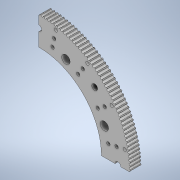
# Autodesk Inventor part: 152ToothBase
Saved by Autodesk Inventor 2020 (Build 240168000, 168)
## iProperties
Created: 2020-01-19
Part Number: 152ToothBase
Material: Generic
Document SubType Name: Modeling
Designer: srini
Density: 1 g/cm^3
Appearance: Default
Author: srini
Autodesk Inventor part; units mm, degrees
ref_plane "YZ Plane" through (0, 0, 0) normal (1, 0, 0) x (0, 1, 0)
ref_plane "XZ Plane" through (0, 0, 0) normal (0, 1, 0) x (-1, 0, 0)
ref_plane "XY Plane" through (0, 0, 0) normal (0, 0, 1) x (1, 0, 0)
sketch "Sketch1" plane through (0, 0, 0) normal (0, 0, 1) x (1, 0, 0)
  circle A0 centre (0, 0) radius 139.485
  dimension "d0" = 278.97
  constraints: 1 centre point, 1 coincident
  measures "d0" diameter of A0
extrude "Extrusion1" add sketch "Sketch1" along normal blind 16
sketch "Sketch2" plane through (0, 0, 16) normal (0, 0, 1) x (1, 0, 0)
  arc A0 (-1.543, 138.9452) -> (1.543, 138.9452) centre (0, 138.9452) ccw
  line L0 (-2.0752, 139.4696) -> (-2.0752, 141.0997)
  line L1 (-2.0752, 141.0997) -> (2.0752, 141.0997)
  line L2 (2.0752, 141.0997) -> (2.0752, 139.4696)
  circle A1 centre (0, 0) radius 139.485 construction
  arc A2 (-1.543, 138.9452) -> (-2.0752, 139.4696) centre (-2.0674, 138.9452) ccw
  arc A3 (2.0752, 139.4696) -> (1.543, 138.9452) centre (2.0674, 138.9452) ccw
  dimension "d3" = 1.543
  dimension "d47" = 2.0828
  constraints: 8 point on circle, 6 end point, 3 centre point, 3 tangent, 2 horizontal alignment, 2 vertical, 1 equal radius, 1 perpendicular, 1 vertical alignment
  measures "d3" radius of A0
extrude "Extrusion2" cut sketch "Sketch2" against normal through all
pattern_circular "Circular Pattern1" count 176 over 360 about axis through (0, 0, 0) along (0, 0, 1) of "Extrusion2"
sketch "Sketch3" plane through (0, 0, 16) normal (0, 0, 1) x (1, 0, 0)
  circle A0 centre (21.06, 105.8758) radius 2.5797
  line L0 (21.06, 105.8758) -> (3.1113, 15.6417) construction
  circle A1 centre (23.5376, 118.3317) radius 2.5797
  circle A2 centre (26.0153, 130.7877) radius 2.5797
  circle A3 centre (-21.06, 105.8758) radius 2.5797
  circle A4 centre (-23.5376, 118.3317) radius 2.5797
  circle A5 centre (-26.0153, 130.7877) radius 2.5797
  circle A6 centre (-59.9738, 89.7571) radius 2.5797
  circle A7 centre (-67.0295, 100.3168) radius 2.5797
  circle A8 centre (-74.0853, 110.8765) radius 2.5797
  circle A9 centre (-89.7571, 59.9738) radius 2.5797
  circle A10 centre (-100.3168, 67.0295) radius 2.5797
  circle A11 centre (-110.8765, 74.0853) radius 2.5797
  circle A12 centre (-105.8758, 21.06) radius 2.5797
  circle A13 centre (-118.3317, 23.5376) radius 2.5797
  circle A14 centre (-130.7877, 26.0153) radius 2.5797
  circle A15 centre (-105.8758, -21.06) radius 2.5797
  circle A16 centre (-118.3317, -23.5376) radius 2.5797
  circle A17 centre (-130.7877, -26.0153) radius 2.5797
  circle A18 centre (-89.7571, -59.9738) radius 2.5797
  circle A19 centre (-100.3168, -67.0295) radius 2.5797
  circle A20 centre (-110.8765, -74.0853) radius 2.5797
  circle A21 centre (-59.9738, -89.7571) radius 2.5797
  circle A22 centre (-67.0295, -100.3168) radius 2.5797
  circle A23 centre (-74.0853, -110.8765) radius 2.5797
  circle A24 centre (-21.06, -105.8758) radius 2.5797
  circle A25 centre (-23.5376, -118.3317) radius 2.5797
  circle A26 centre (-26.0153, -130.7877) radius 2.5797
  circle A27 centre (21.06, -105.8758) radius 2.5797
  circle A28 centre (23.5376, -118.3317) radius 2.5797
  circle A29 centre (26.0153, -130.7877) radius 2.5797
  circle A30 centre (59.9738, -89.7571) radius 2.5797
  circle A31 centre (67.0295, -100.3168) radius 2.5797
  circle A32 centre (74.0853, -110.8765) radius 2.5797
  circle A33 centre (89.7571, -59.9738) radius 2.5797
  circle A34 centre (100.3168, -67.0295) radius 2.5797
  circle A35 centre (110.8765, -74.0853) radius 2.5797
  circle A36 centre (105.8758, -21.06) radius 2.5797
  circle A37 centre (118.3317, -23.5376) radius 2.5797
  circle A38 centre (130.7877, -26.0153) radius 2.5797
  circle A39 centre (105.8758, 21.06) radius 2.5797
  circle A40 centre (118.3317, 23.5376) radius 2.5797
  circle A41 centre (130.7877, 26.0153) radius 2.5797
  circle A42 centre (89.7571, 59.9738) radius 2.5797
  circle A43 centre (100.3168, 67.0295) radius 2.5797
  circle A44 centre (110.8765, 74.0853) radius 2.5797
  circle A45 centre (59.9738, 89.7571) radius 2.5797
  circle A46 centre (67.0295, 100.3168) radius 2.5797
  circle A47 centre (74.0853, 110.8765) radius 2.5797
  circle A48 centre (41.3107, 99.7328) radius 6.35
  line L1 (41.3107, 99.7328) -> (0, 0) construction
  circle A49 centre (-41.3107, 99.7328) radius 6.35
  circle A50 centre (-99.7328, 41.3107) radius 6.35
  circle A51 centre (-99.7328, -41.3107) radius 6.35
  circle A52 centre (-41.3107, -99.7328) radius 6.35
  circle A53 centre (41.3107, -99.7328) radius 6.35
  circle A54 centre (99.7328, -41.3107) radius 6.35
  circle A55 centre (99.7328, 41.3107) radius 6.35
  circle A56 centre (0, 120.269) radius 4.445
  line L2 (0, 120.269) -> (0, 0)
  circle A57 centre (-85.043, 85.043) radius 4.445
  circle A58 centre (-120.269, 0) radius 4.445
  circle A59 centre (-85.043, -85.043) radius 4.445
  circle A60 centre (0, -120.269) radius 4.445
  circle A61 centre (85.043, -85.043) radius 4.445
  circle A62 centre (120.269, 0) radius 4.445
  circle A63 centre (85.043, 85.043) radius 4.445
  line L3 (0, 0) -> (0, 87.7314)
  dimension "d10" = 5.1594
  dimension "d11" = 107.95
  dimension "d14" = 12.7
  dimension "d21" = 360
  dimension "d23" = 12.7
  dimension "d24" = 107.95
  dimension "d25" = 11.25
  dimension "d28" = 360
  dimension "d30" = 120.269
  dimension "d31" = 8.89
  dimension "d33" = 11.25
  dimension "d36" = 360
  dimension "d38" = 11.25
  constraints: 64 centre point, 8 end point, 1 point on line, 1 vertical, 136 other
  measures "d10" diameter of A0
  measures "d11" distance of L1.end L0.start
  measures "d14" distance of L0.start A1.centre
  measures "d23" diameter of A48
  measures "d24" distance of L1.start L1.end
  measures "d25" angle of L1 L0
  measures "d30" distance of L2.start L1.end
  measures "d31" diameter of A56
  measures "d33" angle of L0 L2
  measures "d38" angle of L0 L3
extrude "Extrusion3" cut sketch "Sketch3" against normal through all
sketch "Sketch4" plane through (0, 0, 16) normal (0, 0, 1) x (1, 0, 0)
  circle A0 centre (0, 0) radius 95.25
  dimension "d41" = 190.5
  constraints: 1 centre point, 1 coincident
  measures "d41" diameter of A0
extrude "Extrusion4" cut sketch "Sketch4" against normal through all
sketch "Sketch5" plane through (0, 0, 16) normal (0, 0, 1) x (1, 0, 0)
  line L0 (-193.3483, 162.6718) -> (0, 162.6718)
  line L1 (0, 162.6718) -> (0, 0)
  line L2 (0, 0) -> (-193.3483, 0)
  line L3 (-193.3483, 0) -> (-193.3483, 162.6718)
  line L4 (-193.3483, 0) -> (223.1607, 0)
  line L5 (223.1607, 0) -> (223.1607, -164.8322)
  line L6 (223.1607, -164.8322) -> (-193.3483, -164.8322)
  line L7 (-193.3483, -164.8322) -> (-193.3483, 0)
  constraints: 16 end point, 4 parallel, 2 horizontal, 2 perpendicular
extrude "Extrusion5" cut sketch "Sketch5" against normal through all
sketch "Sketch6" plane through (0, 124.714, 16) normal (-1, 0, 0) x (0, 0, 1)
  line L0 (-28.362, 20.4376) -> (11.0164, 20.4376)
  line L1 (11.0164, 20.4376) -> (11.0164, -44.4017)
  line L2 (11.0164, -44.4017) -> (-28.362, -44.4017)
  line L3 (-28.362, -44.4017) -> (-28.362, 20.4376)
  point P0 (-16, -124.714)
  constraints: 8 end point, 2 parallel, 1 horizontal, 1 perpendicular
extrude "Extrusion6" cut sketch "Sketch6" against normal blind 0.25
body "Solid1"
